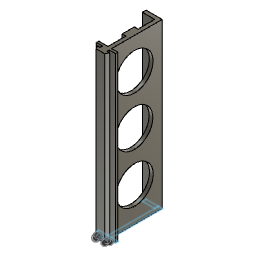
Battery Holder v2 (Autodesk Fusion 360 design; units mm, degrees)
part number: BatteryHolder
Autodesk Fusion 360 part; units mm, degrees
sketch "Sketch1" plane through (0, 0, 0) normal (0, 0, 1) x (1, 0, 0)
  line L0 (-1.5262, 2.741) -> (8.4738, 2.741)
  line L1 (8.4738, 2.741) -> (7, 0.1417)
  line L2 (0.7238, 2.741) -> (6.25, 2.741)
  line L3 (6.25, 2.741) -> (6.25, 4.641)
  line L4 (0.7238, 4.641) -> (0.7238, 2.741)
  line L5 (-1.5262, 2.741) -> (0, 0.1417)
  line L6 (0, 0.1417) -> (7, 0.1417)
  line L7 (0.7238, 4.641) -> (-4.2762, 4.641)
  line L8 (-4.2762, 4.641) -> (-4.2762, 6.641)
  line L9 (6.25, 4.641) -> (11.25, 4.641)
  line L10 (11.25, 4.641) -> (11.25, 6.641)
  line L11 (-4.2762, 6.641) -> (11.25, 6.641)
  line L12 (6.2154, 6.641) -> (3.2154, 6.641)
  line L13 (3.2154, 6.641) -> (3.2154, 47.641)
  line L14 (3.2154, 47.641) -> (6.2154, 47.641)
  line L15 (6.2154, 47.641) -> (6.2154, 6.641)
  line L16 (3.2154, 47.641) -> (-6.7846, 47.641)
  line L17 (-6.7846, 47.641) -> (-6.7846, 44.641)
  line L18 (-6.7846, 44.641) -> (3.2154, 44.641)
  line L19 (3.2154, 44.641) -> (3.2154, 47.641)
  point P0 (0, 0.1417)
  point P1 (7, 0.1417)
  point P2 (8.4738, 2.741)
  point P3 (-1.5262, 2.741)
  point P4 (6.2238, 2.741)
  point P5 (0.7238, 2.741)
  dimension "d1" = 7
  dimension "d2" = 10
  dimension "d4" = 5.5
  dimension "d5" = 2.25
  dimension "d6" = 1.9
  dimension "d53" = 1.9
  dimension "d54" = 5
  dimension "d55" = 2
  dimension "d56" = 5
  dimension "d57" = 2
  dimension "d58" = 3
  dimension "d59" = 41
  dimension "d62" = 10
  dimension "d63" = 3
  constraint horizontal P0 L1.end
  constraint horizontal P2 L0.start
  constraint coincident P3 L0.start
  constraint coincident P2 L0.end
  constraint coincident P1 L1.end
  constraint coincident L0 P4
  constraint coincident L0 P5
  constraint horizontal L2
  constraint vertical L3
  constraint vertical L4
  constraint coincident P5 L2.start
  constraint coincident P0 L5.end
  constraint perpendicular L4 L7
  constraint perpendicular L7 L8
  constraint perpendicular L3 L9
  constraint perpendicular L9 L10
  constraint perpendicular L10 L11
  constraint horizontal L12
  constraint vertical L13
  constraint horizontal L14
  constraint vertical L15
  constraint coincident L11 L12.start
  constraint horizontal L16
  constraint vertical L17
  constraint horizontal L18
  constraint vertical L19
  measures "d1" distance of P0 L1.end
  measures "d2" distance of P2 L0.start
  measures "d4" distance of P4 P5
  measures "d5" distance of P3 P5
  measures "d6" distance of P5 L4.start
  measures "d53" vertical distance of P4 L3.end
  measures "d54" distance of L4.start L7.end
  measures "d55" distance of L7.end L8.end
  measures "d56" distance of L3.end L9.end
  measures "d57" distance of L9.end L10.end
  measures "d58" distance of L12.start L12.end
  measures "d59" distance of L12.start L14.end
  measures "d62" distance of L13.end L16.end
  measures "d63" distance of L13.end L18.end
extrude "Extrude17" add sketch "Sketch1" along normal blind 133
box "BoxPrimitive1" add length 3 width 10 height 3 placed x (0, 0, 1) y (0, 1, 0) z (-1, 0, 0) at (3.2154, 21, 0)
box "BoxPrimitive2" add length 3 width 10 height 3 placed x (0, 0, -1) y (0, -1, 0) z (-1, 0, 0) at (3.2154, 31.1166, 133)
hole "Hole4" at (3.2154, 25.3964, 27.786) direction (1, 0, 0) diameter 30 depth 5 tip angle 180
hole "Hole5" at (3.2154, 25.581, 63.0295) direction (1, 0, 0) diameter 30 depth 5 tip angle 180
hole "Hole6" at (3.2154, 25.5941, 108.2011) direction (1, 0, 0) diameter 30 depth 5 tip angle 180
move_face "MoveFace1" to x (1, 0, 0) y (0, 1, 0) z (0, 0, 1) at (0, -0.4903, 4.7399) 1 faces at (5.2154, 27.0745, 77.955)
move_face "MoveFace2" to x (1, 0, 0) y (0, 1, 0) z (0, 0, 1) at (0, -0.3269, -0.8172) 1 faces at (5.2154, 27.0876, 123.1265)
